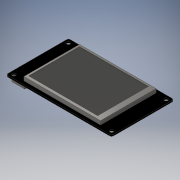
# Autodesk Inventor part: MKF TFT32
Saved by Autodesk Inventor 2018.2 (Build 222227000, 227)
## iProperties
Created: 2018-04-01
Part Number: MKF TFT32
Material: Edelstahl, 440C
Document SubType Name: Modeling
Designer: Till
Density: 7.75 g/cm^3
Appearance: Halbpoliert
Author: Till
Autodesk Inventor part; units mm, degrees
ref_plane "YZ Plane" through (0, 0, 0) normal (1, 0, 0) x (0, 1, 0)
ref_plane "XZ Plane" through (0, 0, 0) normal (0, 1, 0) x (-1, 0, 0)
ref_plane "XY Plane" through (0, 0, 0) normal (0, 0, 1) x (1, 0, 0)
sketch "Skizze1" plane through (0, 0, 0) normal (0, 0, 1) x (1, 0, 0)
  line L0 (-53, 32.5) -> (53, 32.5)
  line L1 (55, 30.5) -> (55, -30.5)
  line L2 (53, -32.5) -> (-53, -32.5)
  line L3 (-55, -30.5) -> (-55, 30.5)
  line L4 (-55, 32.5) -> (55, -32.5) construction
  line L5 (55, 32.5) -> (-55, -32.5) construction
  arc A0 (-53, 32.5) -> (-55, 30.5) centre (-53, 30.5) ccw
  arc A1 (55, 30.5) -> (53, 32.5) centre (53, 30.5) ccw
  arc A2 (53, -32.5) -> (55, -30.5) centre (53, -30.5) ccw
  arc A3 (-55, -30.5) -> (-53, -32.5) centre (-53, -30.5) ccw
  point P0 (0, 0)
  dimension "d0" = 110
  dimension "d1" = 65
  dimension "d2" = 2
  constraints: 12 end point, 8 point on circle, 8 point on line, 8 tangent, 4 centre point, 3 equal radius, 2 midpoint, 2 parallel, 1 horizontal, 1 perpendicular
  measures "d0" distance of L4.end L5.end
  measures "d1" distance of L5.start L4.end
  measures "d2" radius of A0
extrude "Extrusion1" add sketch "Skizze1" along normal blind 1.5
sketch "Skizze2" plane through (0, 0, 1.5) normal (0, 0, 1) x (1, 0, 0)
  circle A0 centre (-51, 28.5) radius 2
  circle A1 centre (-51, -28.5) radius 2
  circle A2 centre (51, -28.5) radius 2
  circle A3 centre (51, 28.5) radius 2
  line L0 (-55, 30.5) -> (-55, -30.5) projected
  line L1 (-53, -32.5) -> (53, -32.5) projected
  point P0 (0, 0)
  dimension "d5" = 4
  dimension "d6" = 4
  dimension "d7" = 4
  dimension "d8" = 4
  dimension "d9" = 102
  dimension "d10" = 102
  dimension "d11" = 57
  dimension "d12" = 57
  dimension "d13" = 4
  dimension "d14" = 4
  dimension "d15" = 4
  dimension "d16" = 4
  constraints: 4 centre point
  measures "d5" diameter of A0
  measures "d6" diameter of A1
  measures "d7" diameter of A2
  measures "d8" diameter of A3
  measures "d9" distance of A3.centre A0.centre
  measures "d10" distance of A2.centre A1.centre
  measures "d11" distance of A3.centre A2.centre
  measures "d12" distance of A1.centre A0.centre
  measures "d13" distance from line of L0 A0.centre
  measures "d14" distance from line of L0 A1.centre
  measures "d15" distance from line of L1 A1.centre
  measures "d16" distance from line of L1 A2.centre
extrude "Extrusion2" cut sketch "Skizze2" against normal up to next
sketch "Skizze3" plane through (0, 0, 1.5) normal (0, 0, 1) x (1, 0, 0)
  line L0 (-40, -29) -> (40, -29)
  line L1 (40, -29) -> (40, 29)
  line L2 (40, 29) -> (-40, 29)
  line L3 (-40, 29) -> (-40, -29)
  line L4 (53, 32.5) -> (-53, 32.5) projected
  line L5 (-55, 30.5) -> (-55, -30.5) projected
  point P0 (0, 0)
  dimension "d19" = 80
  dimension "d20" = 58
  dimension "d21" = 3.5
  dimension "d22" = 15
  constraints: 8 end point, 2 parallel, 1 horizontal, 1 perpendicular
  measures "d19" distance of L2.end L1.end
  measures "d20" distance of L1.end L0.end
  measures "d21" distance between parallel lines of L4 L2
  measures "d22" distance between parallel lines of L5 L3
extrude "Extrusion3" add sketch "Skizze3" along normal blind 4
sketch "Skizze4" plane through (0, 0, 5.5) normal (0, 0, 1) x (1, 0, 0)
  line L0 (-38, -26) -> (34, -26)
  line L1 (34, -26) -> (34, 27)
  line L2 (34, 27) -> (-38, 27)
  line L3 (-38, 27) -> (-38, -26)
  line L4 (-40, 29) -> (-40, -29) projected
  line L5 (40, 29) -> (-40, 29) projected
  point P0 (0, 0)
  dimension "d25" = 72
  dimension "d26" = 53
  dimension "d27" = 2
  dimension "d28" = 2
  constraints: 8 end point, 2 parallel, 1 horizontal, 1 perpendicular
  measures "d25" distance of L2.end L1.end
  measures "d26" distance of L1.end L0.end
  measures "d27" distance between parallel lines of L4 L3
  measures "d28" distance between parallel lines of L5 L2
extrude "Extrusion4" cut sketch "Skizze4" against normal blind 0.3
sketch "Skizze5" plane through (0, 0, 0) normal (0, 0, -1) x (-1, 0, 0)
  line L0 (55, -30.5) -> (55, 30.5) projected
  line L1 (55, -26.5) -> (41.5, -26.5)
  line L2 (41.5, -26.5) -> (41.5, -12)
  line L3 (41.5, -12) -> (55, -12)
  line L4 (55, -12) -> (55, -26.5)
  line L5 (-53, -32.5) -> (53, -32.5) projected
  point P0 (0, 0)
  dimension "d31" = 14.5
  dimension "d32" = 6
  dimension "d33" = 13.5
  constraints: 8 end point, 2 parallel, 1 horizontal, 1 perpendicular, 1 point on line
  measures "d31" distance of L1.end L2.end
  measures "d32" distance between parallel lines of L5 L1
  measures "d33" distance of L2.end L3.end
extrude "Extrusion5" add sketch "Skizze5" along normal blind 8
sketch "Skizze6" plane through (0, 0, 0) normal (0, 0, -1) x (-1, 0, 0)
  line L0 (55, 30.5) -> (55, -30.5) projected
  line L1 (55, 24.5) -> (25, 24.5)
  line L2 (25, 24.5) -> (25, -5.5)
  line L3 (25, -5.5) -> (55, -5.5)
  line L4 (55, -5.5) -> (55, 24.5)
  line L5 (53, 32.5) -> (-53, 32.5) projected
  point P0 (0, 0)
  dimension "d36" = 30
  dimension "d37" = 30
  dimension "d38" = 8
  constraints: 8 end point, 2 parallel, 1 horizontal, 1 perpendicular, 1 point on line
  measures "d36" distance of L3.end L2.end
  measures "d37" distance of L2.end L1.end
  measures "d38" distance between parallel lines of L5 L1
extrude "Extrusion6" add sketch "Skizze6" along normal blind 2.8
